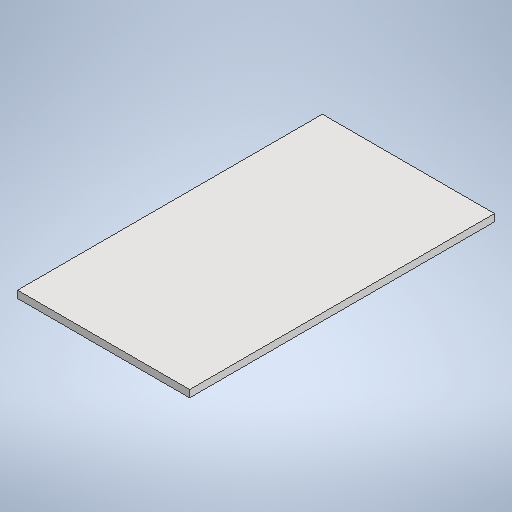
# Autodesk Inventor part: HW-069
Saved by Autodesk Inventor 2025.2 (Build 292293000, 293)
## iProperties
Created: 2026-02-19
Part Number: HW-069
Material: 一般
Document SubType Name: Modeling
Designer: naka6
Density: 1 g/cm^3
Appearance: 既定
Author: naka6
Autodesk Inventor part; units mm, degrees
ref_plane "YZ Plane" through (0, 0, 0) normal (1, 0, 0) x (0, 1, 0)
ref_plane "XZ Plane" through (0, 0, 0) normal (0, 1, 0) x (-1, 0, 0)
ref_plane "XY Plane" through (0, 0, 0) normal (0, 0, 1) x (1, 0, 0)
sketch "スケッチ1" plane through (0, 0, 0) normal (0, 1, 0) x (-1, 0, 0)
  line L0 (12, -21.25) -> (-12, -21.25)
  line L1 (-12, -21.25) -> (-12, 21.25)
  line L2 (-12, 21.25) -> (12, 21.25)
  line L3 (12, 21.25) -> (12, -21.25)
  line L4 (12, -21.25) -> (-12, 21.25) construction
  line L5 (-12, -21.25) -> (12, 21.25) construction
  point P0 (0, 0)
  dimension "d0" = 24
  dimension "d1" = 42.5
  constraints: 12 end point, 2 midpoint, 2 parallel, 1 horizontal, 1 perpendicular
  measures "d0" distance of L1.end L2.end
  measures "d1" distance of L2.end L0.start
extrude "押し出し1" add sketch "スケッチ1" along normal blind 1
